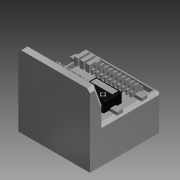
# Autodesk Inventor part: model
Saved by Autodesk Inventor 2014 (Build 180170000, 170)
## iProperties
Created: 2015-02-16
Part Number: model
Material: Générique
Document SubType Name: Modeling
Designer: prazc_000
Density: 1 g/cm^3
Appearance: Galvanized
Author: prazc_000
Autodesk Inventor part; units mm, degrees
ref_plane "YZ Plane" through (0, 0, 0) normal (1, 0, 0) x (0, 1, 0)
ref_plane "XZ Plane" through (0, 0, 0) normal (0, 1, 0) x (-1, 0, 0)
ref_plane "XY Plane" through (0, 0, 0) normal (0, 0, 1) x (1, 0, 0)
sketch "Sketch1" plane through (0, 0, 0) normal (0, 0, 1) x (1, 0, 0)
  line L0 (0, 0) -> (500, 0)
  line L1 (500, 0) -> (500, 500)
  line L2 (500, 500) -> (0, 500)
  line L3 (0, 500) -> (0, 0)
  dimension "d0" = 500
  dimension "d1" = 500
  constraints: 8 end point, 2 parallel, 1 horizontal, 1 perpendicular
  measures "d0" distance between parallel lines of L3 L1
  measures "d1" distance between parallel lines of L0 L2
extrude "Extrusion1" add sketch "Sketch1" along normal blind 500
sketch "Sketch2" plane through (0, 500, 0) normal (0, 1, 0) x (1, 0, 0)
  line L0 (500, 0) -> (500, -500) projected
  line L1 (0, -500) -> (500, -500)
  line L2 (500, -500) -> (500, -250)
  line L3 (500, -250) -> (0, -250)
  line L4 (0, -250) -> (0, -500)
  dimension "d4" = 250
  constraints: 8 end point, 2 parallel, 1 horizontal, 1 midpoint, 1 perpendicular
  measures "d4" distance between parallel lines of L1 L3
extrude "Extrusion2" cut sketch "Sketch2" against normal blind 400
chamfer "Chamfer1" distance 150 angle 20 1 edges at (250, 100, 500) measured on face at (333.3333, 100, 416.6667)
chamfer "Chamfer2" distance 20 angle 45 12 edges at (0, 22.7022, 500) (0, 72.7022, 425) (0, 100, 300) (0, 300, 250) (0, 500, 125) (250, 500, 0) (250, 500, 250) (500, 500, 125) (500, 300, 250) (500, 100, 300) (500, 72.7022, 425) (500, 22.7022, 500)
sketch "Sketch3" plane through (20, 480, 250) normal (0, 0, 1) x (1, 0, 0)
  line L0 (460, 0) -> (460, -380) projected
  line L1 (0, 0) -> (460, 0) projected
  line L2 (0, -380) -> (0, 0) projected
  line L3 (0, -380) -> (460, -380) projected
  line L4 (450, -10) -> (450, -370)
  line L5 (450, -370) -> (10, -370)
  line L6 (10, -370) -> (10, -10)
  line L7 (10, -10) -> (450, -10)
  point P0 (-20, -480)
  dimension "d13" = 10
  constraints: 8 end point, 3 other
  measures "d13" distance between parallel lines of L7 L1
extrude "Extrusion3" cut sketch "Sketch3" against normal blind 30 contours L4 L5 L6 L7
sketch "Sketch4" plane through (0, 0, 0) normal (-1, 0, 0) x (0, 0, 1)
  line L0 (250, 100) -> (250, 480) projected
  line L1 (250, 400) -> (270, 400)
  line L2 (270, 400) -> (270, 360)
  line L3 (270, 360) -> (250, 360)
  line L4 (250, 360) -> (250, 400)
  line L5 (250, 230) -> (270, 230)
  line L6 (270, 230) -> (270, 190)
  line L7 (270, 190) -> (250, 190)
  line L8 (250, 190) -> (250, 230)
  dimension "d16" = 20
  dimension "d17" = 20
  dimension "d18" = 40
  dimension "d19" = 40
  dimension "d20" = 80
  dimension "d21" = 130
  constraints: 16 end point, 4 parallel, 2 horizontal, 2 perpendicular, 2 point on line
  measures "d16" distance between parallel lines of L2 L4
  measures "d17" distance between parallel lines of L6 L8
  measures "d18" distance between parallel lines of L3 L1
  measures "d19" distance between parallel lines of L7 L5
  measures "d20" distance from line of L1 L0.end
  measures "d21" distance between parallel lines of L5 L3
extrude "Extrusion4" add sketch "Sketch4" against normal up to surface (500 mm away)
sketch "Sketch5" plane through (0, 190, 270) normal (0, 0, 1) x (1, 0, 0)
  line L0 (500, 0) -> (500, 40) projected
  line L1 (0, 0) -> (0, 40) projected
  line L2 (270, 85) -> (450, 85)
  line L3 (450, 85) -> (450, -45)
  line L4 (450, -45) -> (270, -45)
  line L5 (270, -45) -> (270, 85)
  line L6 (270, 20) -> (450, 20) construction
  line L7 (0, 20) -> (500, 20) construction
  point P0 (0, -190)
  dimension "d24" = 130
  dimension "d25" = 180
  dimension "d26" = 50
  constraints: 12 end point, 4 midpoint, 2 parallel, 1 collinear, 1 horizontal, 1 perpendicular
  measures "d24" distance between parallel lines of L4 L2
  measures "d25" distance between parallel lines of L5 L3
  measures "d26" distance between parallel lines of L0 L3
extrude "Extrusion5" add sketch "Sketch5" along normal blind 60
sketch "Sketch6" plane through (0, 190, 270) normal (0, 0, -1) x (-1, 0, 0)
  line L0 (-270, 40) -> (-450, 40) projected
  line L1 (-270, 40) -> (-270, 85) projected
  line L2 (-270, 85) -> (-450, 85) projected
  line L3 (-450, 85) -> (-450, 40) projected
  line L4 (-270, 0) -> (-450, 0) projected
  line L5 (-450, 0) -> (-450, -45) projected
  line L6 (-450, -45) -> (-270, -45) projected
  line L7 (-270, -45) -> (-270, 0) projected
  point P0 (0, -190)
extrude "Extrusion6" add sketch "Sketch6" along normal blind 10
chamfer "Chamfer3" distance 5 angle 45 8 edges at (270, 275, 295) (360, 275, 330) (450, 275, 295) (270, 210, 330) (360, 145, 330) (450, 210, 330) (450, 145, 295) (270, 145, 295)
sketch "Sketch7" plane through (0, 190, 330) normal (0, 0, 1) x (1, 0, 0)
  line L0 (445, -40) -> (275, -40) projected
  line L1 (445, 80) -> (445, -40) projected
  line L2 (275, -40) -> (275, 80) projected
  line L3 (382.5736, -3.7868) -> (425, -3.7868) construction
  line L4 (403.7868, 17.4264) -> (403.7868, -25) construction
  line L5 (393.1802, 6.8198) -> (393.1802, -14.3934)
  line L6 (393.1802, -14.3934) -> (414.3934, -14.3934)
  line L7 (414.3934, -14.3934) -> (414.3934, 6.8198)
  line L8 (393.1802, 6.8198) -> (414.3934, 6.8198)
  line L9 (394.1802, 7.8198) -> (413.3934, 7.8198)
  line L10 (415.3934, -13.3934) -> (415.3934, 5.8198)
  line L11 (392.1802, 5.8198) -> (392.1802, -13.3934)
  line L12 (394.1802, -15.3934) -> (413.3934, -15.3934)
  line L13 (425, -3.7868) -> (415.3934, 5.8198)
  line L14 (413.3934, 7.8198) -> (403.7868, 17.4264)
  line L15 (403.7868, -25) -> (413.3934, -15.3934)
  line L16 (415.3934, -13.3934) -> (425, -3.7868)
  line L17 (382.5736, -3.7868) -> (392.1802, -13.3934)
  line L18 (394.1802, -15.3934) -> (403.7868, -25)
  line L19 (403.7868, 17.4264) -> (394.1802, 7.8198)
  line L20 (392.1802, 5.8198) -> (382.5736, -3.7868)
  point P0 (0, -190)
  dimension "d41" = 1
  dimension "d42" = 1
  dimension "d43" = 1
  dimension "d44" = 1
  dimension "d45" = 15
  dimension "d46" = 20
  constraints: 36 end point, 15 parallel, 5 perpendicular, 4 collinear, 1 horizontal
  measures "d41" distance between parallel lines of L8 L9
  measures "d42" distance between parallel lines of L5 L11
  measures "d43" distance between parallel lines of L10 L7
  measures "d44" distance between parallel lines of L12 L6
  measures "d45" distance from line of L0 L4.end
  measures "d46" distance from line of L1 L3.end
extrude "Extrusion7" add sketch "Sketch7" along normal blind 5 contours L19 L14 L9 | L10 L13 L16 | L11 L17 L20 | L12 L15 L18
sketch "Sketch8" plane through (0, 190, 330) normal (0, 0, 1) x (1, 0, 0)
  line L0 (445, 80) -> (445, -40) projected
  line L1 (275, 80) -> (445, 80) projected
  line L2 (275, -40) -> (275, 80) projected
  line L3 (285, 70) -> (435, 70)
  line L4 (435, 70) -> (435, 30)
  line L5 (435, 30) -> (285, 30)
  line L6 (285, 30) -> (285, 70)
  point P0 (0, -190)
  dimension "d49" = 10
  dimension "d50" = 10
  dimension "d51" = 10
  dimension "d52" = 40
  constraints: 8 end point, 2 parallel, 1 horizontal, 1 perpendicular
  measures "d49" distance between parallel lines of L2 L6
  measures "d50" distance between parallel lines of L0 L4
  measures "d51" distance between parallel lines of L3 L1
  measures "d52" distance between parallel lines of L5 L3
extrude "Extrusion8" add sketch "Sketch8" along normal blind 3
sketch "Sketch9" plane through (0, 190, 270) normal (0, 0, 1) x (1, 0, 0)
  line L0 (0, 0) -> (0, 40) projected
  line L1 (0, 0) -> (270, 0) projected
  line L2 (50, 63) -> (68, 63)
  line L3 (68, 63) -> (68, -23)
  line L4 (68, -23) -> (50, -23)
  line L5 (50, -23) -> (50, 63)
  line L6 (50, 20) -> (68, 20) construction
  line L7 (0, 20) -> (146.78, 20) construction
  point P0 (0, -190)
  dimension "d55" = 18
  dimension "d56" = 86
  dimension "d57" = 50
  constraints: 12 end point, 3 midpoint, 3 parallel, 1 collinear, 1 horizontal, 1 perpendicular
  measures "d55" distance between parallel lines of L5 L3
  measures "d56" distance between parallel lines of L4 L2
  measures "d57" distance between parallel lines of L0 L5
extrude "Extrusion9" add sketch "Sketch9" along normal blind 60
sketch "Sketch10" plane through (0, 190, 330) normal (0, 0, 1) x (1, 0, 0)
  line L0 (68, 63) -> (50, 63) projected
  line L1 (68, -23) -> (68, 63) projected
  line L2 (50, 63) -> (68, 63)
  line L3 (68, 63) -> (68, 43)
  line L4 (68, 43) -> (50, 43)
  line L5 (50, 43) -> (50, 63)
  line L6 (50, -23) -> (68, -23)
  line L7 (68, -23) -> (68, -3)
  line L8 (68, -3) -> (50, -3)
  line L9 (50, -3) -> (50, -23)
  point P0 (0, -190)
  dimension "d60" = 20
  dimension "d61" = 20
  dimension "d62" = 46
  constraints: 16 end point, 4 parallel, 2 horizontal, 2 perpendicular, 2 point on line
  measures "d60" distance between parallel lines of L6 L8
  measures "d61" distance between parallel lines of L0 L4
  measures "d62" distance between parallel lines of L8 L4
extrude "Extrusion10" cut sketch "Sketch10" against normal blind 25
sketch "Sketch11" plane through (50, 230, 270) normal (-1, 0, 0) x (0, 0, 1)
  line L0 (60, 3) -> (35, 3) projected
  line L1 (60, 3) -> (60, -43) projected
  line L2 (60, -17) -> (68.1008, -10.0211)
  line L3 (68.1008, -10.0211) -> (71.3643, -13.8092)
  line L4 (71.3643, -13.8092) -> (60, -23.5996)
  point P0 (-270, -230)
  dimension "d65" = 15
  dimension "d66" = 5
  dimension "d67" = 20
  constraints: 6 end point, 2 point on line, 1 parallel, 1 perpendicular
  measures "d65" distance from line of L4.end L3
  measures "d66" distance between parallel lines of L4 L2
  measures "d67" distance from line of L0 L2.start
extrude "Extrusion11" add sketch "Sketch11" against normal up to surface (18 mm away)
sketch "Sketch12" plane through (0, 190, 270) normal (0, 0, -1) x (-1, 0, 0)
  line L0 (-50, 40) -> (-68, 40) projected
  line L1 (-50, 40) -> (-50, 63) projected
  line L2 (-50, 63) -> (-68, 63) projected
  line L3 (-68, 63) -> (-68, 40) projected
  line L4 (-50, 0) -> (-68, 0) projected
  line L5 (-68, 0) -> (-68, -23) projected
  line L6 (-68, -23) -> (-50, -23) projected
  line L7 (-50, -23) -> (-50, 0) projected
  point P0 (0, -190)
extrude "Extrusion12" add sketch "Sketch12" along normal blind 10
chamfer "Chamfer4" distance 2 angle 45 18 edges at (50, 223, 330) (50, 233, 317.5) (50, 243, 305) (68, 243, 305) (59, 253, 305) (68, 233, 317.5) (68, 223, 330) (50, 196.7002, 330) (68, 196.7002, 330) (59, 187, 330) (68, 177, 305) (50, 177, 305) (59, 167, 305) (59, 233, 330) (59, 219.9789, 338.1008) (50, 218.0849, 339.7325) (59, 216.1908, 341.3643) (68, 218.0849, 339.7325)
pattern_linear "Rectangular Pattern1" count 5 spacing 40 along (1, 0, 0) of "Extrusion9", "Extrusion10", "Chamfer4", "Extrusion11", "Extrusion12"
sketch "Sketch13" plane through (0, 360, 270) normal (0, 0, 1) x (1, 0, 0)
  line L0 (500, 0) -> (500, 40) projected
  line L1 (0, 0) -> (0, 40) projected
  line L2 (440, 62.5) -> (450, 62.5)
  line L3 (450, 62.5) -> (450, -22.5)
  line L4 (450, -22.5) -> (440, -22.5)
  line L5 (440, -22.5) -> (440, 62.5)
  line L6 (440, 20) -> (450, 20) construction
  line L7 (0, 20) -> (500, 20) construction
  point P0 (0, -360)
  dimension "d78" = 85
  dimension "d79" = 10
  dimension "d80" = 50
  constraints: 12 end point, 4 midpoint, 2 parallel, 1 collinear, 1 horizontal, 1 perpendicular
  measures "d78" distance between parallel lines of L4 L2
  measures "d79" distance between parallel lines of L5 L3
  measures "d80" distance between parallel lines of L0 L3
extrude "Extrusion13" add sketch "Sketch13" along normal blind 50
sketch "Sketch14" plane through (0, 360, 320) normal (0, 0, 1) x (1, 0, 0)
  line L0 (440, -22.5) -> (450, -22.5) projected
  line L1 (450, -22.5) -> (450, 62.5) projected
  line L2 (440, 62.5) -> (450, 62.5)
  line L3 (450, 62.5) -> (450, 42.5)
  line L4 (450, 42.5) -> (440, 42.5)
  line L5 (440, 42.5) -> (440, 62.5)
  line L6 (440, -22.5) -> (450, -22.5)
  line L7 (450, -22.5) -> (450, -2.5)
  line L8 (450, -2.5) -> (440, -2.5)
  line L9 (440, -2.5) -> (440, -22.5)
  point P0 (0, -360)
  dimension "d83" = 20
  dimension "d84" = 20
  constraints: 16 end point, 4 parallel, 2 horizontal, 2 perpendicular, 2 point on line
  measures "d83" distance between parallel lines of L2 L4
  measures "d84" distance between parallel lines of L0 L8
extrude "Extrusion14" cut sketch "Sketch14" against normal blind 30
chamfer "Chamfer5" distance 10 angle 45 2 edges at (445, 402.5, 320) (445, 357.5, 320)
chamfer "Chamfer6" distance 5 angle 45 2 edges at (445, 422.5, 290) (445, 337.5, 290)
sketch "Sketch15" plane through (0, 360, 270) normal (0, 0, -1) x (-1, 0, 0)
  line L0 (-440, 40) -> (-450, 40) projected
  line L1 (-440, 40) -> (-440, 62.5) projected
  line L2 (-440, 62.5) -> (-450, 62.5) projected
  line L3 (-450, 62.5) -> (-450, 40) projected
  line L4 (-440, 0) -> (-450, 0) projected
  line L5 (-450, 0) -> (-450, -22.5) projected
  line L6 (-450, -22.5) -> (-440, -22.5) projected
  line L7 (-440, -22.5) -> (-440, 0) projected
  point P0 (0, -360)
extrude "Extrusion15" add sketch "Sketch15" along normal blind 10
pattern_linear "Rectangular Pattern2" count 10 spacing 30 along (-1, 0, 0) of "Extrusion13", "Extrusion15", "Chamfer5", "Extrusion14"
sketch "Sketch16" plane through (0, 360, 270) normal (0, 0, 1) x (1, 0, 0)
  line L0 (0, 0) -> (0, 40) projected
  line L1 (50, 62.5) -> (75, 62.5)
  line L2 (75, 62.5) -> (75, -22.5)
  line L3 (75, -22.5) -> (50, -22.5)
  line L4 (50, -22.5) -> (50, 62.5)
  point P0 (0, -360)
  point P1 (50, 20)
  point P2 (0, 20)
  dimension "d98" = 85
  dimension "d99" = 25
  dimension "d100" = 50
  constraints: 8 end point, 2 midpoint, 2 parallel, 1 horizontal, 1 horizontal alignment, 1 perpendicular
  measures "d98" distance between parallel lines of L3 L1
  measures "d99" distance between parallel lines of L2 L4
  measures "d100" distance between parallel lines of L0 L4
extrude "Extrusion16" add sketch "Sketch16" along normal blind 40
sketch "Sketch17" plane through (0, 360, 270) normal (0, 0, -1) x (-1, 0, 0)
  line L0 (-50, 40) -> (-75, 40) projected
  line L1 (-50, 40) -> (-50, 62.5) projected
  line L2 (-50, 62.5) -> (-75, 62.5) projected
  line L3 (-75, 62.5) -> (-75, 40) projected
  line L4 (-50, 0) -> (-75, 0) projected
  line L5 (-75, 0) -> (-75, -22.5) projected
  line L6 (-75, -22.5) -> (-50, -22.5) projected
  line L7 (-50, -22.5) -> (-50, 0) projected
  point P0 (0, -360)
extrude "Extrusion17" add sketch "Sketch17" along normal blind 10
chamfer "Chamfer7" distance 2 angle 45 4 edges at (62.5, 337.5, 310) (75, 380, 310) (62.5, 422.5, 310) (50, 380, 310)
pattern_linear "Rectangular Pattern3" count 3 spacing 40 along (1, 0, 0) of "Extrusion16", "Chamfer7", "Extrusion17"
body "Solid1"
